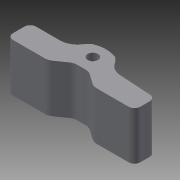
# Autodesk Inventor part: FelixOriginalLever
Saved by Autodesk Inventor 2015 SP1 (Build 190203100, 203)
## iProperties
Created: 2014-12-15
Part Number: FelixOriginalLever
Material: Generic
Document SubType Name: Modeling
Designer: Jack
Density: 1 g/cm^3
Appearance: Default
Author: Jack
Autodesk Inventor part; units mm, degrees
ref_plane "YZ Plane" through (0, 0, 0) normal (1, 0, 0) x (0, 1, 0)
ref_plane "XZ Plane" through (0, 0, 0) normal (0, 1, 0) x (-1, 0, 0)
ref_plane "XY Plane" through (0, 0, 0) normal (0, 0, 1) x (1, 0, 0)
sketch "Sketch1" plane through (0, 0, 0) normal (0, 0, 1) x (1, 0, 0)
  line L0 (0, 0) -> (51.4289, 0) construction
  line L1 (51.4289, 0) -> (51.4289, -25.9828) construction
  line L2 (51.4289, -25.9828) -> (0, -25.9828) construction
  line L3 (0, -25.9828) -> (0, 0) construction
  circle A0 centre (24.9, -9.85) radius 2
  line L4 (1.6, -19.55) -> (1.6, -10.65)
  line L5 (1.6, -10.65) -> (13.1, -10.65)
  line L6 (1.6, -19.55) -> (17.4, -19.55)
  line L7 (17.4, -19.55) -> (23.2, -15.45)
  line L8 (23.2, -15.45) -> (29, -15.45)
  line L9 (29, -15.45) -> (34.8, -19.55)
  line L10 (34.8, -19.55) -> (50.6, -19.55)
  line L11 (50.6, -19.55) -> (50.6, -11.55)
  line L12 (50.6, -11.55) -> (36.1, -10.6377)
  arc A1 (31.1534, -7.6382) -> (29.195, -5.6092) centre (25.0705, -11.55) ccw
  arc A2 (20.6046, -5.6092) -> (18.6461, -7.6382) centre (24.7291, -11.55) ccw
  arc A3 (31.1534, -7.6382) -> (36.1, -10.6377) centre (36.4916, -4.4135) ccw
  arc A4 (13.1, -10.65) -> (18.6461, -7.6382) centre (13.1, -4.0375) ccw
  ellipse E0 centre (24.9, -20.05) end of major axis (24.9008, -35.35) minor radius 13 (29.195, -5.6092) -> (20.6046, -5.6092) ccw
  dimension "d45" = 13
  dimension "d46" = 15.3
  dimension "d22" = 4
  dimension "d35" = 0.5
  dimension "d36" = 1.6
  dimension "d37" = 10.65
  dimension "d38" = 8.9
  dimension "d39" = 3.6
  dimension "d47" = 8
  dimension "d51" = 17.4
  dimension "d52" = 25.7
  dimension "d53" = 9.7
  dimension "d54" = 11.5
  dimension "d55" = 14.5
  dimension "d57" = 0.3414
  dimension "d59" = 5.8
  dimension "d61" = 4.1
  dimension "d63" = 15.8
  dimension "d64" = 15.8
  dimension "d66" = 8
  dimension "d72" = 0.1705
  dimension "d76" = 7.2322
  dimension "d77" = 6.2366
  constraints: 20 end point, 8 point on circle, 5 centre point, 4 horizontal alignment, 2 horizontal, 2 perpendicular, 2 point on line, 2 tangent, 2 vertical, 1 coincident, 1 equal length, 1 equal radius, 1 parallel, 1 vertical alignment, 6 other
  measures "d22" diameter of A0
  measures "d35" distance from line of L6 point (24.9, -20.05)
  measures "d36" distance from line of point (0, 0) L4
  measures "d37" distance from line of point (0, 0) L5
  measures "d38" distance between parallel lines of L5 L6
  measures "d39" angle of L10 L12
  measures "d47" distance of L10.end L11.end
  measures "d51" distance of L6.end L9.end
  measures "d52" distance from line of L11 point (24.9, -20.05)
  measures "d53" distance from line of L10 A0.centre
  measures "d54" distance from line of L4 L5.end
  measures "d55" horizontal distance of L11.end L12.end
  measures "d57" distance of A1.centre A2.centre
  measures "d59" distance of L7.end L8.end
  measures "d61" distance between parallel lines of L10 L8
  measures "d63" distance from line of L4 L6.end
  measures "d64" distance from line of L11 L9.end
  measures "d66" distance from line of L10 A1.centre
  measures "d72" horizontal distance of A0.centre A1.centre
  measures "d76" radius of A2
  measures "d77" radius of A3
extrude "Extrusion1" add sketch "Sketch1" along normal blind 18.5
fillet "Fillet1" radius 2.25 4 edges at (1.6, -10.65, 9.25) (1.6, -19.55, 9.25) (50.6, -11.55, 9.25) (50.6, -19.55, 9.25)
fillet "Fillet2" radius 4 4 edges at (23.2, -15.45, 9.25) (29, -15.45, 9.25) (34.8, -19.55, 9.25) (17.4, -19.55, 9.25)
body "Solid1"
